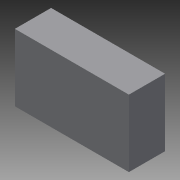
# Autodesk Inventor part: conrad_Strapubox_2028
Saved by Autodesk Inventor 2014 SP1 (Build 180222100, 222)
## iProperties
Created: 2015-08-04
Part Number: conrad_Strapubox_2028
Material: Générique
Document SubType Name: Modeling
Designer: astralien3000
Density: 1 g/cm^3
Appearance: Par défaut
Author: astralien3000
Autodesk Inventor part; units mm, degrees
ref_plane "YZ Plane" through (0, 0, 0) normal (1, 0, 0) x (0, 1, 0)
ref_plane "XZ Plane" through (0, 0, 0) normal (0, 1, 0) x (-1, 0, 0)
ref_plane "XY Plane" through (0, 0, 0) normal (0, 0, 1) x (1, 0, 0)
sketch "Esquisse1" plane through (0, 0, 0) normal (0, 1, 0) x (-1, 0, 0)
  line L0 (0, 0) -> (85, 0)
  line L1 (85, 0) -> (85, 50)
  line L2 (85, 50) -> (0, 50)
  line L3 (0, 50) -> (0, 0)
  dimension "d0" = 85
  dimension "d1" = 50
  constraints: 8 end point, 2 parallel, 1 horizontal, 1 perpendicular
  measures "d0" distance of L1.end L2.end
  measures "d1" distance of L0.end L1.end
extrude "Extrusion1" add sketch "Esquisse1" along normal blind 27
sketch "Esquisse2" plane through (0, 27, 0) normal (0, 1, 0) x (1, 0, 0)
  line L0 (0, 0) -> (-85, 0) projected
  line L1 (-85, 0) -> (-85, -50) projected
  line L2 (-85, -50) -> (0, -50) projected
  line L3 (0, -50) -> (0, 0) projected
  line L4 (-82.5, -2.5) -> (-78.5532, -2.5)
  line L5 (-2.5, -2.5) -> (-2.5, -5.8909)
  line L6 (-2.5, -47.5) -> (-78.5532, -47.5)
  line L7 (-82.5, -47.5) -> (-82.5, -44.1091)
  line L8 (-82.5, -2.5) -> (-2.5, -47.5) construction
  line L9 (-2.5, -2.5) -> (-82.5, -47.5) construction
  circle A0 centre (-81.5, -3.0625) radius 2
  arc A1 (-78.8853, -4.5333) -> (-78.5532, -2.5) centre (-81.5, -3.0625) ccw
  line L10 (-42.5, -25) -> (-42.5, -2.5) construction
  line L11 (-42.5, -25) -> (-82.5, -25) construction
  circle A2 centre (-3.5, -3.0625) radius 2
  arc A3 (-6.1147, -4.5333) -> (-2.5, -5.8909) centre (-3.5, -3.0625) ccw
  circle A4 centre (-81.5, -46.9375) radius 2
  arc A5 (-78.5532, -47.5) -> (-82.5, -44.1091) centre (-81.5, -46.9375) ccw
  circle A6 centre (-3.5, -46.9375) radius 2
  arc A7 (-6.1147, -45.4667) -> (-6.4468, -47.5) centre (-3.5, -46.9375) ccw
  arc A8 (-82.5, -5.8909) -> (-78.8853, -4.5333) centre (-81.5, -3.0625) ccw
  arc A9 (-78.5532, -2.5) -> (-82.5, -5.8909) centre (-81.5, -3.0625) ccw
  arc A10 (-6.4468, -2.5) -> (-6.1147, -4.5333) centre (-3.5, -3.0625) ccw
  arc A11 (-2.5, -5.8909) -> (-6.4468, -2.5) centre (-3.5, -3.0625) ccw
  arc A12 (-2.5, -44.1091) -> (-6.1147, -45.4667) centre (-3.5, -46.9375) ccw
  arc A13 (-6.4468, -47.5) -> (-2.5, -44.1091) centre (-3.5, -46.9375) ccw
  arc A14 (-82.5, -44.1091) -> (-78.5532, -47.5) centre (-81.5, -46.9375) ccw
  line L12 (-78.5532, -47.5) -> (-82.5, -47.5)
  line L13 (-82.5, -44.1091) -> (-82.5, -2.5)
  line L14 (-42.5, -2.5) -> (-6.4468, -2.5)
  line L15 (-78.5532, -2.5) -> (-42.5, -2.5)
  line L16 (-6.4468, -2.5) -> (-2.5, -2.5)
  line L17 (-2.5, -5.8909) -> (-2.5, -25)
  line L18 (-2.5, -44.1091) -> (-2.5, -47.5)
  line L19 (-2.5, -25) -> (-2.5, -44.1091)
  dimension "d4" = 2.5
  dimension "d5" = 2.5
  dimension "d6" = 2.5
  dimension "d7" = 2.5
  dimension "d8" = 4
  dimension "d9" = 6
  dimension "d10" = 1
  constraints: 32 end point, 22 point on circle, 16 parallel, 16 perpendicular, 15 centre point, 10 point on line, 6 symmetric about line, 4 coincident, 4 horizontal, 1 midpoint, 6 other
  measures "d4" distance between parallel lines of L0 L4
  measures "d5" distance between parallel lines of L2 L6
  measures "d6" distance between parallel lines of L1 L7
  measures "d7" distance between parallel lines of L3 L5
  measures "d8" diameter of A0
  measures "d9" diameter of A1
  measures "d10" distance from line of L7 A0.centre
extrude "Extrusion2" cut sketch "Esquisse2" against normal blind 25 contours L13 A0 L4 | L4 A0 L13 | L15 L14 A10 A3 L17 L19 A12 A7 L6 A5 L13 A8 A1 | A4 L12 L7 | L7 L12 A4 | L16 L5 A2 | A2 L5 L16 | A6 L18 L6 | L6 L18 A6
equation "\"d5\" = d4"
equation "\"d6\" = d4"
equation "\"d7\" = d4"
